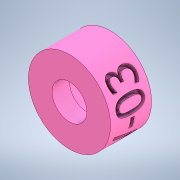
# Autodesk Inventor part: brakeLockSpacer
Saved by Autodesk Inventor 2021.1 (Build 251245000, 245)
## iProperties
Created: 2020-08-18
Part Number: brakeLockSpacer
Material: Polycarbonate, Smoke
Document SubType Name: Modeling
Designer: robst
Density: 1.2 g/cm^3
Appearance: Pink
Author: robst
Autodesk Inventor part; units mm, degrees
ref_plane "XZ Plane" through (0, 0, 0) normal (0, 1, 0) x (-1, 0, 0)
ref_plane "XY Plane" through (0, 0, 0) normal (0, 0, 1) x (1, 0, 0)
sketch "Sketch1" plane through (0, 0, 0) normal (0, 0, 1) x (1, 0, 0)
  circle A0 centre (0, 0) radius 8.0645
  circle A1 centre (0, 0) radius 19.05
  dimension "d0" = 16.129
  dimension "d1" = 38.1
  constraints: 2 centre point, 2 coincident
  measures "d0" diameter of A0
  measures "d1" diameter of A1
extrude "Extrusion1" add sketch "Sketch1" against normal blind 19.05
sketch "Sketch3" plane through (0, 0, 0) normal (1, 0, 0) x (0, 1, 0)
  line L0 (0, 0) -> (0, -127) construction
  line L1 (-8.0645, -19.05) -> (-8.0645, 0) construction
  line L2 (-19.05, -19.05) -> (19.05, -19.05) construction
  line L3 (8.0645, -19.05) -> (8.0645, 0) construction
  line L4 (8.0645, -19.05) -> (8.0645, -8.0515)
  line L5 (8.0645, -8.0515) -> (14.4145, -19.05)
  line L6 (8.0645, -19.05) -> (22.7292, -19.05)
  dimension "d8" = 30
  dimension "d10" = 6.35
  constraints: 8 end point, 1 parallel, 1 point on line, 2 other
  measures "d8" angle of L5 L3
  measures "d10" distance of L5.end L3.start
revolve "Revolution1" cut sketch "Sketch3" angle 360 about axis through (0, 0, 0) along (0, 0, -1)
ref_plane "Work Plane1" through (19.05, 0, 0) normal (1, 0, 0) x (0, 1, 0)
sketch "Sketch9" plane through (19.05, 0, 0) normal (1, 0, 0) x (0, 1, 0)
  line L0 (19.05, 0) -> (19.05, -19.05) construction
  line L1 (19.05, -9.525) -> (-19.05, -9.525) construction
  line L2 (-19.05, 0) -> (-19.05, -19.05) construction
  line L3 (-7.4152, -3.175) -> (-11.7892, -15.875)
  line L4 (-11.7892, -15.875) -> (-13.6108, -15.875)
  line L5 (-13.6108, -15.875) -> (-17.9848, -3.175)
  line L6 (-17.9848, -3.175) -> (-16.1735, -3.175)
  line L7 (-16.1735, -3.175) -> (-12.6537, -13.724)
  line L8 (-12.6537, -13.724) -> (-9.1339, -3.175)
  line L9 (-9.1339, -3.175) -> (-7.4152, -3.175)
  line L10 (-1.765, -11.0893) -> (-6.5713, -11.0893)
  line L11 (-6.5713, -11.0893) -> (-6.5713, -9.5456)
  line L12 (-6.5713, -9.5456) -> (-1.765, -9.5456)
  line L13 (-1.765, -9.5456) -> (-1.765, -11.0893)
  spline S0 degree 2 poles (7.8269, -9.525) (7.8269, -12.9419) (5.8406, -16.1426) (3.7719, -16.1426) knots 0 0 0 1 2 2 2
  spline S1 degree 2 poles (3.7719, -16.1426) (1.6724, -16.1426) (-0.2933, -12.8801) (-0.2933, -9.5353) knots 0 0 0 1 2 2 2
  spline S2 degree 2 poles (-0.2933, -9.5353) (-0.2933, -6.0979) (1.693, -2.9177) (3.7719, -2.9177) knots 0 0 0 1 2 2 2
  spline S3 degree 2 poles (3.7719, -2.9177) (5.8611, -2.9177) (7.8269, -6.2111) (7.8269, -9.525) knots 0 0 0 1 2 2 2
  spline S4 degree 2 poles (5.645, -13.3947) (5.892, -12.7669) (6.0979, -10.8321) (6.0979, -9.525) knots 0 0 0 1 2 2 2
  spline S5 degree 2 poles (6.0979, -9.525) (6.0979, -8.2179) (5.892, -6.2934) (5.6347, -5.645) knots 0 0 0 1 2 2 2
  spline S6 degree 2 poles (5.6347, -5.645) (5.3774, -4.9966) (4.4821, -4.3277) (3.7719, -4.3277) knots 0 0 0 1 2 2 2
  spline S7 degree 2 poles (3.7719, -4.3277) (3.0618, -4.3277) (2.1458, -4.9966) (1.8782, -5.6656) knots 0 0 0 1 2 2 2
  spline S8 degree 2 poles (1.8782, -5.6656) (1.6209, -6.314) (1.4357, -8.29) (1.4357, -9.5353) knots 0 0 0 1 2 2 2
  spline S9 degree 2 poles (1.4357, -9.5353) (1.4357, -10.8732) (1.6004, -12.664) (1.868, -13.3638) knots 0 0 0 1 2 2 2
  spline S10 degree 2 poles (1.868, -13.3638) (2.115, -14.0225) (3.0309, -14.7326) (3.7719, -14.7326) knots 0 0 0 1 2 2 2
  spline S11 degree 2 poles (3.7719, -14.7326) (4.4718, -14.7326) (5.3877, -14.0637) (5.645, -13.3947) knots 0 0 0 1 2 2 2
  spline S12 degree 2 poles (12.8801, -4.3791) (12.417, -4.3791) (11.501, -4.6056) (11.0585, -4.7805) knots 0 0 0 1 2 2 2
  spline S13 degree 2 poles (11.0585, -4.7805) (10.6468, -4.9555) (10.0396, -5.326) (9.8029, -5.4906) knots 0 0 0 1 2 2 2
  line L14 (9.8029, -5.4906) -> (9.7, -5.4906)
  line L15 (9.7, -5.4906) -> (9.7, -3.6896)
  spline S14 degree 2 poles (9.7, -3.6896) (10.2557, -3.3911) (12.1597, -2.9074) (13.0139, -2.9074) knots 0 0 0 1 2 2 2
  spline S15 degree 2 poles (13.0139, -2.9074) (13.8784, -2.9074) (15.1649, -3.2573) (15.6897, -3.6278) knots 0 0 0 1 2 2 2
  spline S16 degree 2 poles (15.6897, -3.6278) (16.2455, -4.0292) (16.8218, -5.1922) (16.8218, -5.9744) knots 0 0 0 1 2 2 2
  spline S17 degree 2 poles (16.8218, -5.9744) (16.8218, -7.0241) (15.4427, -8.609) (14.4753, -8.8149) knots 0 0 0 1 2 2 2
  line L16 (14.4753, -8.8149) -> (14.4753, -8.9384)
  spline S18 degree 2 poles (14.4753, -8.9384) (14.8767, -9.0207) (15.7927, -9.3912) (16.1838, -9.7617) knots 0 0 0 1 2 2 2
  spline S19 degree 2 poles (16.1838, -9.7617) (16.5748, -10.1219) (17.0688, -11.2746) (17.0688, -12.1082) knots 0 0 0 1 2 2 2
  spline S20 degree 2 poles (17.0688, -12.1082) (17.0688, -12.9624) (16.4822, -14.4136) (15.947, -14.9693) knots 0 0 0 1 2 2 2
  spline S21 degree 2 poles (15.947, -14.9693) (15.3913, -15.5457) (13.8167, -16.1426) (12.8184, -16.1426) knots 0 0 0 1 2 2 2
  spline S22 degree 2 poles (12.8184, -16.1426) (11.8612, -16.1426) (9.9881, -15.6795) (9.35, -15.3604) knots 0 0 0 1 2 2 2
  line L17 (9.35, -15.3604) -> (9.35, -13.5594)
  line L18 (9.35, -13.5594) -> (9.4735, -13.5594)
  spline S23 degree 2 poles (9.4735, -13.5594) (10.0087, -13.9504) (11.8201, -14.6709) (12.7154, -14.6709) knots 0 0 0 1 2 2 2
  spline S24 degree 2 poles (12.7154, -14.6709) (13.2403, -14.6709) (14.2901, -14.3415) (14.64, -13.9607) knots 0 0 0 1 2 2 2
  spline S25 degree 2 poles (14.64, -13.9607) (14.9796, -13.5799) (15.3398, -12.6743) (15.3398, -11.9847) knots 0 0 0 1 2 2 2
  spline S26 degree 2 poles (15.3398, -11.9847) (15.3398, -11.2952) (14.9385, -10.3998) (14.5782, -10.1425) knots 0 0 0 1 2 2 2
  spline S27 degree 2 poles (14.5782, -10.1425) (14.218, -9.8852) (13.2403, -9.6897) (12.664, -9.6897) knots 0 0 0 1 2 2 2
  line L19 (12.664, -9.6897) -> (11.9436, -9.6897)
  line L20 (11.9436, -9.6897) -> (11.9436, -8.2797)
  line L21 (11.9436, -8.2797) -> (12.5096, -8.2797)
  spline S28 degree 2 poles (12.5096, -8.2797) (13.652, -8.2797) (15.0928, -7.1888) (15.0928, -6.1493) knots 0 0 0 1 2 2 2
  spline S29 degree 2 poles (15.0928, -6.1493) (15.0928, -5.6656) (14.7223, -4.9761) (14.4239, -4.7702) knots 0 0 0 1 2 2 2
  spline S30 degree 2 poles (14.4239, -4.7702) (14.1048, -4.5541) (13.3226, -4.3791) (12.8801, -4.3791) knots 0 0 0 1 2 2 2
  point P0 (0, 0)
  constraints: 2 end point, 2 midpoint, 1 horizontal
emboss "Emboss1" sketch "Sketch9" operation cut depth 2.54 direction (-1, 0, 0) wrap yes faces at (18.9882, -1.5329, -12.7)
equation "\"d0\" = innerDiameter"
equation "\"d1\" = outsideDiameter"
equation "\"d8\" = brakeHandle"
equation "\"d10\" = heightOfBrake"
equation "\"brakeHandle\" = 30deg"
equation "\"innerDiameter\" = 16.129"
equation "\"heightOfBrake\" = 6.35"
equation "\"outsideDiameter\" = 38.1"
equation "\"d36\" = 0.5 * outsideDiameter"
body "Solid1"
